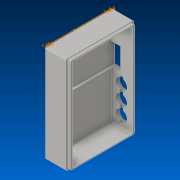
# Autodesk Inventor part: Bottom
Saved by Autodesk Inventor 2016 (Build 200138000, 138)
## iProperties
Created: 2015-08-21
Part Number: Bottom
Material: Generic
Document SubType Name: Modeling
Designer: Moffitt
Density: 1 g/cm^3
Appearance: Default
Author: Moffitt
Autodesk Inventor part; units mm, degrees
ref_plane "YZ Plane" through (0, 0, 0) normal (1, 0, 0) x (0, 1, 0)
ref_plane "XZ Plane" through (0, 0, 0) normal (0, 1, 0) x (-1, 0, 0)
ref_plane "XY Plane" through (0, 0, 0) normal (0, 0, 1) x (1, 0, 0)
sketch "Very Bottom" plane through (0, 0, 0) normal (1, 0, 0) x (0, 1, 0)
  line L0 (98.706, 61.2459) -> (-101.294, 61.2459)
  line L1 (-101.294, 61.2459) -> (-101.294, -78.7541)
  line L2 (-101.294, -78.7541) -> (98.706, -78.7541)
  line L3 (98.706, -78.7541) -> (98.706, 61.2459)
  point P0 (0, 0)
  dimension "d4" = 140
  dimension "d5" = 200
  constraints: 8 end point, 2 parallel, 1 horizontal, 1 perpendicular
  measures "d4" distance of L2.end L0.start
  measures "d5" distance of L1.end L2.end
extrude "Extrusion1" add sketch "Very Bottom" along normal blind 10
sketch "Walls A" plane through (10, 0, 0) normal (1, 0, 0) x (0, 0, -1)
  line L0 (-53.2459, 94.706) -> (70.7541, 94.706)
  line L1 (70.7541, 94.706) -> (70.7541, -97.294)
  line L2 (70.7541, -97.294) -> (-53.2459, -97.294)
  line L3 (-53.2459, -97.294) -> (-53.2459, 94.706)
  line L4 (78.7541, 98.706) -> (-61.2459, 98.706) projected
  line L5 (-61.2459, -101.294) -> (78.7541, -101.294) projected
  line L6 (-61.2459, 98.706) -> (-61.2459, -101.294) projected
  line L7 (78.7541, -101.294) -> (78.7541, 98.706) projected
  point P0 (0, 0)
  dimension "d6" = 4
  dimension "d7" = 4
  dimension "d8" = 8
  dimension "d9" = 8
  constraints: 8 end point, 2 parallel, 1 horizontal, 1 perpendicular
  measures "d6" distance between parallel lines of L4 L0
  measures "d7" distance between parallel lines of L5 L2
  measures "d8" distance between parallel lines of L3 L6
  measures "d9" distance between parallel lines of L7 L1
extrude "Walls" add sketch "Walls A" along normal blind 40
sketch "Meeting Lip" plane through (50, 0, 0) normal (1, 0, 0) x (0, 0, -1)
  line L0 (-57.2459, 96.706) -> (74.7541, 96.706)
  line L1 (74.7541, 96.706) -> (74.7541, -99.294)
  line L2 (74.7541, -99.294) -> (-57.2459, -99.294)
  line L3 (-57.2459, -99.294) -> (-57.2459, 96.706)
  line L4 (-61.2459, 98.706) -> (-61.2459, -101.294) projected
  line L5 (78.7541, -101.294) -> (78.7541, 98.706) projected
  line L6 (-61.2459, -101.294) -> (78.7541, -101.294) projected
  line L7 (78.7541, 98.706) -> (-61.2459, 98.706) projected
  point P0 (0, 0)
  dimension "d18" = 4
  dimension "d19" = 4
  dimension "d20" = 2
  dimension "d21" = 2
  constraints: 8 end point, 2 parallel, 1 horizontal, 1 perpendicular
  measures "d18" distance between parallel lines of L4 L3
  measures "d19" distance between parallel lines of L5 L1
  measures "d20" distance between parallel lines of L6 L2
  measures "d21" distance between parallel lines of L0 L7
extrude "Top Lip" cut sketch "Meeting Lip" against normal blind 5.5
sketch "Back Panel" plane through (0, -101.294, -78.7541) normal (0, 0, -1) x (-1, 0, 0)
  circle A0 centre (-26.5, 24) radius 12
  circle A1 centre (-26.5, 52) radius 12
  circle A2 centre (-26.5, 80) radius 12
  line L0 (0, 0) -> (-44.5, 0) projected
  line L1 (-44.5, 200) -> (-44.5, 0) projected
  line L2 (-10, 4) -> (-10, 196) projected
  line L3 (-10, 103.5669) -> (-25, 103.5669)
  line L4 (-25, 103.5669) -> (-25, 147.5669)
  line L5 (-25, 147.5669) -> (-10, 147.5669)
  line L6 (-10, 147.5669) -> (-10, 103.5669)
  line L7 (-10, 147.5669) -> (-6, 147.5669)
  line L8 (-6, 147.5669) -> (-6, 103.5669)
  line L9 (-6, 103.5669) -> (-10, 103.5669)
  line L10 (-10, 103.5669) -> (-10, 147.5669)
  point P0 (0, 101.294)
  dimension "d24" = 24
  dimension "d25" = 24
  dimension "d26" = 24
  dimension "d27" = 28
  dimension "d28" = 28
  dimension "d29" = 24
  dimension "d30" = 18
  dimension "d31" = 0
  dimension "d32" = 0
  dimension "d33" = 44
  dimension "d34" = 15
  dimension "d52" = 4
  constraints: 16 end point, 4 parallel, 3 centre point, 2 horizontal, 2 perpendicular, 1 point on line
  measures "d24" diameter of A2
  measures "d25" diameter of A1
  measures "d26" diameter of A0
  measures "d27" distance of A1.centre A0.centre
  measures "d28" distance of A2.centre A1.centre
  measures "d29" distance from line of L0 A0.centre
  measures "d30" distance from line of L1 A2.centre
  measures "d31" horizontal distance of A2.centre A1.centre
  measures "d32" horizontal distance of A1.centre A0.centre
  measures "d33" distance of L3.end L4.end
  measures "d34" distance of L4.end L5.end
  measures "d52" distance of L5.end L7.end
extrude "Back Panel Cutouts" cut sketch "Back Panel" against normal blind 8
chamfer "Chamfer1" distance 1 angle 45 4 edges at (15.5, 46.273, -78.7541) (25, 24.273, -78.7541) (15.5, 2.273, -78.7541) (6, 24.273, -78.7541)
fillet "Fillet1" radius 3 12 edges at (22.25, 98.706, -78.7541) (0, -1.294, -78.7541) (22.25, -101.294, -78.7541) (0, -101.294, -8.7541) (22.25, -101.294, 61.2459) (0, -1.294, 61.2459) (22.25, 98.706, 61.2459) (30, 94.706, 53.2459) (30, 94.706, -70.7541) (30, -97.294, -70.7541) (30, -97.294, 53.2459) (0, 98.706, -8.7541)
fillet "Fillet2" radius 3 4 edges at (47.25, 96.706, 57.2459) (47.25, 96.706, -74.7541) (47.25, -99.294, -74.7541) (47.25, -99.294, 57.2459)
sketch "Sketch5" plane through (10, 0, 0) normal (1, 0, 0) x (0, 0, -1)
  line L0 (77.7541, 2.273) -> (70.7541, 2.273) projected
  line L1 (77.7541, 2.273) -> (-22.2459, 2.273)
  line L2 (-22.2459, 2.273) -> (-22.2459, 46.273)
  line L3 (-22.2459, 46.273) -> (77.7541, 46.273)
  line L4 (77.7541, 46.273) -> (77.7541, 2.273)
  line L5 (70.7541, 91.706) -> (70.7541, -94.294) projected
  line L6 (-14.2459, 46.273) -> (70.7541, 46.273)
  line L7 (70.7541, 46.273) -> (70.7541, 50.273)
  line L8 (70.7541, 50.273) -> (-14.2459, 50.273)
  line L9 (-14.2459, 50.273) -> (-14.2459, 46.273)
  point P0 (0, 0)
  dimension "d43" = 100
  dimension "d47" = 8
  dimension "d48" = 4
  constraints: 16 end point, 4 parallel, 2 horizontal, 2 perpendicular, 2 point on line
  measures "d43" distance of L2.end L3.end
  measures "d47" distance from line of L2.end L9
  measures "d48" distance of L8.end L6.start
extrude "PCB Slot" cut sketch "Sketch5" against normal blind 4
chamfer "Chamfer2" distance 4 angle 45 1 edges at (10, 50.273, -28.2541)
fillet "Fillet4" radius 3 9 edges at (10, 93.8273, 52.3672) (10, -1.294, 53.2459) (10, -96.4153, 52.3672) (10, -97.294, -8.7541) (10, -96.4153, -69.8754) (10, -46.0105, -70.7541) (10, 93.8273, -69.8754) (10, 72.9894, -70.7541) (10, 94.706, -8.7541)
sketch "Sketch7" plane through (6, 46.273, -70.7541) normal (0, 0, 1) x (1, 0, 0)
  line L0 (24.5, -138.5669) -> (16.5, -138.5669)
  line L1 (16.5, -138.5669) -> (16.5, -52.5669)
  line L2 (16.5, -52.5669) -> (24.5, -52.5669)
  line L3 (24.5, -52.5669) -> (24.5, -138.5669)
  circle A0 centre (20.5, -123.5669) radius 12 projected
  circle A1 centre (20.5, -67.5669) radius 12 projected
  point P0 (-6, -46.273)
  dimension "d56" = 8
  dimension "d57" = 15
  dimension "d58" = 15
  dimension "d59" = 4
  dimension "d60" = 4
  constraints: 8 end point, 2 parallel, 1 horizontal, 1 perpendicular
  measures "d56" distance of L0.start L0.end
  measures "d57" distance from line of L0 A0.centre
  measures "d58" distance from line of L2 A1.centre
  measures "d59" distance from line of L3 A1.centre
  measures "d60" distance from line of A1.centre L1
extrude "Extrusion7" cut sketch "Sketch7" against normal blind 5 contours L0 L1 A0 L3 | A0 L1 L3 | A0 L1 A1 L3 | A1 L1 L3 | A1 L1 L2 L3
chamfer "Chamfer3" distance 0.5 angle 45 16 edges at (30.5, -9.9803, -73.2541) (30.5, -6.294, -73.2541) (22.5, -6.294, -73.2541) (22.5, -9.9803, -73.2541) (30.5, -32.6077, -73.2541) (30.5, -37.9803, -73.2541) (22.5, -32.6077, -73.2541) (22.5, -37.9803, -73.2541) (30.5, -60.6077, -73.2541) (22.5, -60.6077, -73.2541) (30.5, -65.9803, -73.2541) (22.5, -65.9803, -73.2541) (30.5, -88.6077, -73.2541) (30.5, -92.294, -73.2541) (22.5, -92.294, -73.2541) (22.5, -88.6077, -73.2541)
sketch "Sketch9" plane through (3, 98.706, -75.7541) normal (0, 1, 0) x (1, 0, 0)
  line L0 (-3, 0) -> (-3, -134) projected
  line L1 (-3, -132.5) -> (-1.5, -132.5)
  line L2 (-1.5, -132.5) -> (-1.5, -130.5)
  line L3 (-1.5, -130.5) -> (-3, -130.5)
  line L4 (-3, -130.5) -> (-3, -132.5)
  line L5 (-3, -128.5) -> (-1.5, -128.5)
  line L6 (-1.5, -128.5) -> (-1.5, -126.5)
  line L7 (-1.5, -126.5) -> (-3, -126.5)
  line L8 (-3, -126.5) -> (-3, -128.5)
  line L9 (-3, -1.5) -> (-1.5, -1.5)
  line L10 (-1.5, -1.5) -> (-1.5, -3.5)
  line L11 (-1.5, -3.5) -> (-3, -3.5)
  line L12 (-3, -3.5) -> (-3, -1.5)
  line L13 (-3, -5.5) -> (-1.5, -5.5)
  line L14 (-1.5, -5.5) -> (-1.5, -7.5)
  line L15 (-1.5, -7.5) -> (-3, -7.5)
  line L16 (-3, -7.5) -> (-3, -5.5)
  point P0 (-3, -75.7541)
  dimension "d66" = 1.5
  dimension "d67" = 1.5
  dimension "d68" = 2
  dimension "d69" = 2
  dimension "d70" = 2
  dimension "d71" = 2
  dimension "d72" = 2
  dimension "d73" = 1.5
  dimension "d74" = 2
  dimension "d75" = 1.5
  dimension "d76" = 1.5
  constraints: 32 end point, 8 parallel, 5 point on line, 4 horizontal, 4 perpendicular
  measures "d66" distance of L14.end L15.end
  measures "d67" distance of L10.end L11.end
  measures "d68" distance of L9.end L10.end
  measures "d69" distance of L13.end L14.end
  measures "d70" distance between parallel lines of L11 L13
  measures "d71" distance of L1.end L2.end
  measures "d72" distance of L5.end L6.end
  measures "d73" distance from line of L0.end L1
  measures "d74" distance between parallel lines of L5 L3
  measures "d75" distance of L6.end L7.end
  measures "d76" distance from line of L0.start L9
body "Solid1"
